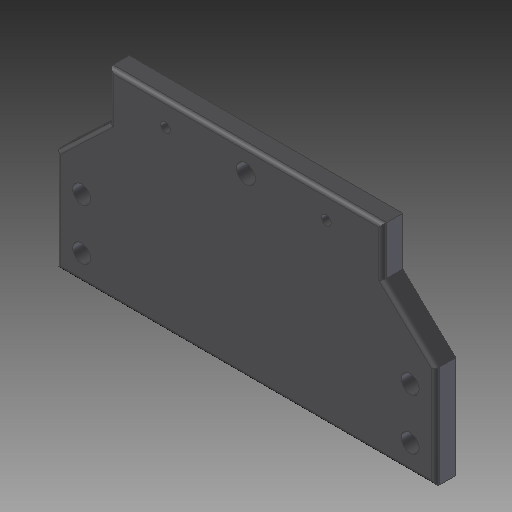
# Autodesk Inventor part: 1136_RU Top Plate_V1
Saved by Autodesk Inventor 2020 (Build 240168000, 168)
## iProperties
Created: 2019-05-13
Part Number: 1136_RU Top Plate_V1
Material: Aluminum
Document SubType Name: Modeling
Designer: e22ma
Density: 2.7 g/cm^3
Appearance: Satin
Mass: 445.599 g
Surface Area: 398.429 cm^2
Volume: 165.037 cm^3
Author: e22ma
Autodesk Inventor part; units mm, degrees
ref_plane "YZ Plane" through (0, 0, 0) normal (1, 0, 0) x (0, 1, 0)
ref_plane "XZ Plane" through (0, 0, 0) normal (0, 1, 0) x (-1, 0, 0)
ref_plane "Work Plane4" through (164.3995, -80, 0) normal (0, 0, 1) x (1, 0, 0)
sketch "Sketch1" plane through (164.3995, -80, 0) normal (0, 0, 1) x (1, 0, 0)
  circle A0 centre (-12.7, -38.1) radius 4.5 projected
  circle A1 centre (-12.7, -12.7) radius 4.5 projected
  circle A2 centre (-176.0991, -12.7) radius 4.5 projected
  circle A3 centre (-176.0991, -38.1) radius 4.5 projected
  line L0 (0, -50.8) -> (-188.7991, -50.8) projected
  line L1 (0, 0) -> (0, -50.8) projected
  line L2 (-188.7991, 0) -> (0, 0) projected
  line L3 (-188.7991, 0) -> (-188.7991, -50.8) projected
  circle A4 centre (-94.3995, 37) radius 4.7625
  circle A5 centre (-134.3995, 37) radius 2.489
  circle A6 centre (-54.3995, 37) radius 2.489
  line L4 (-26.3995, 25) -> (-162.3995, 25)
  line L5 (-26.3995, 49) -> (-26.3995, 25)
  line L6 (-162.3995, 49) -> (-26.3995, 49)
  line L7 (-162.3995, 25) -> (-162.3995, 49)
  line L8 (-26.3995, 25) -> (0, 0)
  line L9 (-162.3995, 25) -> (-188.7991, 0)
  point P0 (-94.3995, 0)
  dimension "d5" = 136
  dimension "d6" = 24
  dimension "d7" = 28
  dimension "d8" = 12
  dimension "d9" = 12
  dimension "d10" = 68
  dimension "d11" = 40
  dimension "d12" = 12
  dimension "d13" = 25
  dimension "d14" = 9.525
  dimension "d15" = 4.978
  dimension "d16" = 4.978
  constraints: 12 end point, 3 centre point, 2 horizontal, 2 vertical, 1 midpoint, 1 vertical alignment
  measures "d5" distance of L6.start L5.start
  measures "d6" distance of L5.start L4.start
  measures "d7" distance from line of L5 A6.centre
  measures "d8" distance from line of L6 A6.centre
  measures "d9" distance from line of L6 A4.centre
  measures "d10" distance from line of L5 A4.centre
  measures "d11" distance of A4.centre A5.centre
  measures "d12" distance from line of L6 A5.centre
  measures "d13" distance between parallel lines of L2 L4
  measures "d14" diameter of A4
  measures "d15" diameter of A5
  measures "d16" diameter of A6
extrude "Extrusion1" add sketch "Sketch1" along normal blind 10
fillet "Fillet3" radius 2 8 edges at (70, -130.8, 10) (164.3995, -105.4, 10) (151.1998, -67.5, 10) (138, -43, 10) (70, -31, 10) (2, -43, 10) (-11.1998, -67.5, 10) (-24.3995, -105.4, 10)
body "Solid1"
